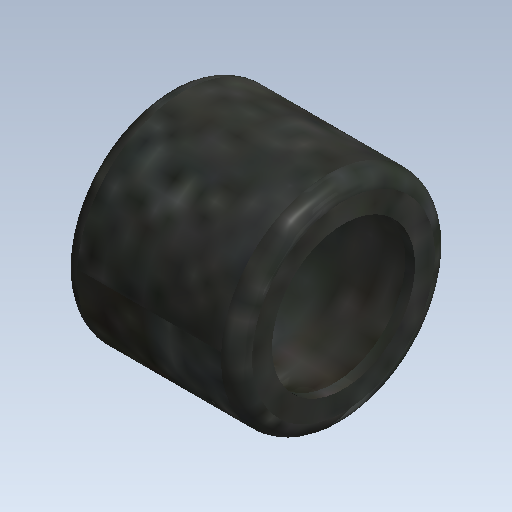
# Autodesk Inventor part: HK0709FMSH
Saved by Autodesk Inventor 2021 (Build 250183000, 183)
## iProperties
Part Number: HK0709FMSH
Material: Steel
Catalog Web Link: www.cadenas.de
Description: Needle Roller Shell Bearings open-ended SH-
Vendor: NTN
Document SubType Name: Modeling
Designer: partserver
Manufacturer: NTN
Mass: 1.38603 g
Surface Area: 7.30394 cm^2
Volume: 0.176564 cm^3
Density: 7.85 g/cm^3
Appearance: Plate
Category: PARTsolutions
Company: NTN
PSOL_IDENT_0: {$CADENAS_DATA\23d-libs\ntn\needle_roler_bearings\needle_roller_shell_bearings_open_ended.prj},196 {
PSOL_IDENT_1: VTYP=3D},{NB=HK0709FMSH},{LINA=HK0709FMSH},{NN=Needle Roller Shell Bearings open-ended SH},{DATE=26.
PSOL_IDENT_2: 11.2019 01:59:50},{GEOMDATE=26.11.2019 00:10:00},{VERSION=},{LINEID=50},{WBVAR=},{WBNUMERIC=}  {NB=H
PSOL_IDENT_3: K0709FMSH},{LINA=HK0709FMSH},{KT=DUMMY},{FW=7},{D=11.0},{C=9},{ORDER=HK0709FM},{CR=3150},{COR=2930},
PSOL_IDENT_4: {CRF=320},{CORF=299},{LSG=23000},{LSO=34000},{MASS=0.0025},{IT=-},{RT=1.6},{VER=1},{T=0.500},{DW=1.5
PSOL_IDENT_5: 00},{LW=5.000},{NR=10.000},{CID=7.750},{CD=9.250},{CW=7.600},{SD=7.350}
NB: HK0709FMSH
NN: Needle Roller Shell Bearings open-ended SH
NBSYN: $ORDER.SH
LINA: HK0709FMSH
CATALOG: NTN Corporation
FW: 7
D: 11
C: 9
ORDER: HK0709FM
CR: 3150
COR: 2930
CRF: 320
CORF: 299
LSG: 23000
LSO: 34000
MASS: 0.0025
IT: -
SUPPLIER: NTN
ARTICLENO: HK0709FMSH
BOMINFO: HK0709FMSH
CREATOR: CADENAS GmbH
Title: HK0709FMSH
Author: Cadenas PARTsolutions
Autodesk Inventor part; units mm, degrees
sketch "Sketch_1" plane through (0, 0, 0) normal (0, 0, 1) x (1, 0, 0)
  line L0 (9, 0) -> (0, 0)
  line L1 (0, 3.675) -> (0.5, 3.675)
  line L2 (0.5, 3.675) -> (0.5, 4.7)
  arc A0 (0.8, 5) -> (0.5, 4.7) centre (0.8, 4.7) ccw
  line L3 (0.8, 5) -> (8.2, 5)
  arc A1 (8.5, 4.7) -> (8.2, 5) centre (8.2, 4.7) ccw
  line L4 (8.5, 4.7) -> (8.5, 3.675)
  line L5 (8.5, 3.675) -> (9, 3.675)
  line L6 (9, 3.675) -> (9, 4.7)
  arc A2 (9, 4.7) -> (8.2, 5.5) centre (8.2, 4.7) ccw
  line L7 (8.2, 5.5) -> (0.8, 5.5)
  arc A3 (0.8, 5.5) -> (0, 4.7) centre (0.8, 4.7) ccw
  line L8 (0, 4.7) -> (0, 3.675)
  constraints: 18 end point, 8 point on circle, 4 centre point
revolve "Revolution1" add sketch "Sketch_1" angle 360 about axis through (9, 0, 0) along (1, 0, 0)
ref_plane "IP_1_XY" through (0, 0, 0) normal (1, 0, 0) x (0, 0, -1)
ref_plane "IP_1_YZ" through (0, 0, 0) normal (0, 0, -1) x (0, 1, 0)
ref_plane "IP_1_ZX" through (0, 0, 0) normal (0, 1, 0) x (1, 0, 0)
ref_plane "IP_5_XY" through (4.5, 0, 0) normal (1, 0, 0) x (0, 0, -1)
ref_plane "IP_5_YZ" through (4.5, 0, 0) normal (0, 0, -1) x (0, 1, 0)
ref_plane "IP_5_ZX" through (4.5, 0, 0) normal (0, 1, 0) x (1, 0, 0)
ref_plane "IP_6_XY" through (6.35, 0, 0) normal (1, 0, 0) x (0, 0, -1)
ref_plane "IP_6_YZ" through (6.35, 0, 0) normal (0, 0, -1) x (0, 1, 0)
ref_plane "IP_6_ZX" through (6.35, 0, 0) normal (0, 1, 0) x (1, 0, 0)
body "Solid1"
